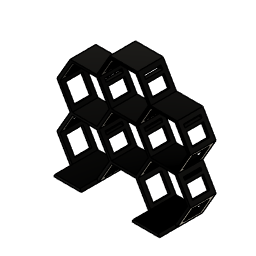
Estande v1 (Autodesk Fusion 360 design; units mm, degrees)
Autodesk Fusion 360 part; units mm, degrees
sketch "Sketch1" plane through (0, 0, 0) normal (0, 1, 0) x (1, 0, 0)
  line L0 (28.8675, 0) -> (14.4338, 25)
  line L1 (14.4338, 25) -> (-14.4338, 25)
  line L2 (-14.4338, 25) -> (-28.8675, 0)
  line L3 (-28.8675, 0) -> (-14.4338, -25)
  line L4 (-14.4338, -25) -> (14.4338, -25)
  line L5 (14.4338, -25) -> (28.8675, 0)
  line L6 (-125, -81) -> (125, -81)
  line L7 (125, -81) -> (125, 67)
  line L8 (125, 67) -> (-125, 67)
  line L9 (-125, 67) -> (-125, -81)
  line L10 (60.3331, 1.5) -> (74.7669, 26.5)
  line L11 (74.7669, 26.5) -> (60.3331, 51.5)
  line L12 (60.3331, 51.5) -> (31.4656, 51.5)
  line L13 (31.4656, 51.5) -> (17.0318, 26.5)
  line L14 (17.0318, 26.5) -> (31.4656, 1.5)
  line L15 (31.4656, 1.5) -> (60.3331, 1.5)
  line L16 (0, 0) -> (45.8993, 26.5) construction
  line L17 (0, 0) -> (0, 25) construction
  line L18 (14.4338, 78) -> (-14.4338, 78)
  line L19 (-14.4338, 78) -> (-28.8675, 53)
  line L20 (-28.8675, 53) -> (-14.4338, 28)
  line L21 (-14.4338, 28) -> (14.4338, 28)
  line L22 (28.8675, 53) -> (14.4338, 78)
  line L23 (14.4338, 28) -> (28.8675, 53)
  line L24 (-60.3331, 51.5) -> (-74.7669, 26.5)
  line L25 (-74.7669, 26.5) -> (-60.3331, 1.5)
  line L26 (-60.3331, 1.5) -> (-31.4656, 1.5)
  line L27 (-31.4656, 1.5) -> (-17.0318, 26.5)
  line L28 (-31.4656, 51.5) -> (-60.3331, 51.5)
  line L29 (-17.0318, 26.5) -> (-31.4656, 51.5)
  line L30 (-74.7669, -26.5) -> (-60.3331, -51.5)
  line L31 (-60.3331, -51.5) -> (-31.4656, -51.5)
  line L32 (-31.4656, -51.5) -> (-17.0318, -26.5)
  line L33 (-17.0318, -26.5) -> (-31.4656, -1.5)
  line L34 (-60.3331, -1.5) -> (-74.7669, -26.5)
  line L35 (-31.4656, -1.5) -> (-60.3331, -1.5)
  line L36 (-14.4338, -78) -> (14.4338, -78)
  line L37 (14.4338, -78) -> (28.8675, -53)
  line L38 (28.8675, -53) -> (14.4338, -28)
  line L39 (14.4338, -28) -> (-14.4338, -28)
  line L40 (-28.8675, -53) -> (-14.4338, -78)
  line L41 (-14.4338, -28) -> (-28.8675, -53)
  line L42 (60.3331, -51.5) -> (74.7669, -26.5)
  line L43 (74.7669, -26.5) -> (60.3331, -1.5)
  line L44 (60.3331, -1.5) -> (31.4656, -1.5)
  line L45 (31.4656, -1.5) -> (17.0318, -26.5)
  line L46 (31.4656, -51.5) -> (60.3331, -51.5)
  line L47 (17.0318, -26.5) -> (31.4656, -51.5)
  line L48 (0, -78) -> (0, -81) construction
  line L49 (125, 54.5) -> (-125, 54.5)
  line L50 (-62.0652, 54.5) -> (-78.231, 26.5)
  line L51 (-78.231, 26.5) -> (-62.7147, -0.375)
  line L52 (-62.7147, -0.375) -> (-78.231, -27.25)
  line L53 (-78.231, -27.25) -> (-62.7147, -54.125)
  line L54 (-62.7147, -54.125) -> (-31.6821, -54.125)
  line L55 (-31.6821, -54.125) -> (-16.1658, -81)
  line L56 (62.0652, 54.5) -> (78.231, 26.5)
  line L57 (78.231, 26.5) -> (62.7147, -0.375)
  line L58 (62.7147, -0.375) -> (78.231, -27.25)
  line L59 (78.231, -27.25) -> (62.7147, -54.125)
  line L60 (62.7147, -54.125) -> (31.6821, -54.125)
  line L61 (31.6821, -54.125) -> (16.1658, -81)
  line L62 (-28.8675, 53) -> (-29.7335, 54.5)
  line L63 (28.8675, 53) -> (29.7335, 54.5)
  point P0 (45.8993, 26.5)
  dimension "d3" = 50
  dimension "d4" = 60
  dimension "d5" = 3
  dimension "d6" = 148
  dimension "d7" = 250
  dimension "d9" = 360
  dimension "d10" = 3
  dimension "d11" = 3
  dimension "d12" = 3
  dimension "d14" = 3
  constraint coincident L16.start L17.start
  constraint horizontal L6
  constraint perpendicular L6 L7
  constraint perpendicular L7 L8
  constraint vertical L9
  constraint horizontal L4
  constraint horizontal L15
  constraint equal L0 L14
  constraint coincident P0 L16.end
  constraint midpoint L1 L17.end
  constraint midpoint L36 L48.start
  constraint midpoint L6 L48.end
  constraint vertical L48
  constraint coincident L7 L49.start
  constraint coincident L9 L49.end
  constraint perpendicular L9 L49
  constraint coincident L49 L50.start
  constraint parallel L49 L54
  constraint coincident L6 L55.end
  constraint parallel L53 L55
  constraint parallel L40 L55
  constraint parallel L34 L52
  constraint parallel L25 L51
  constraint parallel L24 L50
  constraint equal L54 L55
  constraint equal L53 L54
  constraint equal L52 L53
  constraint equal L51 L52
  constraint symmetric L17 L50.start L56.start
  constraint symmetric L17 L50.end L56.end
  constraint symmetric L17 L51.end L57.end
  constraint symmetric L17 L52.end L58.end
  constraint symmetric L17 L53.end L59.end
  constraint symmetric L17 L54.end L60.end
  constraint symmetric L17 L55.end L61.end
  constraint coincident L49 L62.end
  constraint parallel L20 L62
  constraint coincident L49 L63.end
  constraint parallel L23 L63
  measures "d3" distance of L1 L4
  measures "d4" angle of L16 L17
  measures "d5" distance of L0 L14
  measures "d6" distance of L6 L8
  measures "d7" distance of L6.start L6.end
  measures "d10" distance of L6 L36
  measures "d11" distance of L28 L49
  measures "d12" distance of L24 L50
  measures "d14" distance of L25 L51
extrude "Extrude1" add sketch "Sketch1" against normal blind 30 contours L6 L20 L21 L23 L49 L50 L51 L52 L53 L54 L55 L56 L57 L58 L59 L60 L61 L62 L63
sketch "Sketch2" plane through (70.4728, 0, 40.6875) normal (0.866025, 0, 0.5) x (0, 1, 0)
  line L0 (0, -15.5163) -> (0, 15.5163)
  line L1 (0, 15.5163) -> (-30, 15.5163)
  line L2 (-30, 15.5163) -> (-30, -15.5163)
  line L3 (-30, -15.5163) -> (0, -15.5163)
  line L4 (-25, -10.5163) -> (-5, -10.5163)
  line L5 (-5, -10.5163) -> (-5, 10.5163)
  line L6 (-5, 10.5163) -> (-25, 10.5163)
  line L7 (-25, 10.5163) -> (-25, -10.5163)
  line L8 (0, 31.0326) -> (0, 62.0652)
  line L9 (0, 62.0652) -> (-30, 62.0652)
  line L10 (-30, 62.0652) -> (-30, 31.0326)
  line L11 (-30, 31.0326) -> (0, 31.0326)
  line L12 (0, -62.0652) -> (0, -31.0326)
  line L13 (0, -31.0326) -> (-30, -31.0326)
  line L14 (-30, -31.0326) -> (-30, -62.0652)
  line L15 (-30, -62.0652) -> (0, -62.0652)
  line L16 (-25, -57.0652) -> (-5, -57.0652)
  line L17 (-5, -57.0652) -> (-5, -36.0326)
  line L18 (-5, -36.0326) -> (-25, -36.0326)
  line L19 (-25, -36.0326) -> (-25, -57.0652)
  line L20 (-25, 36.0326) -> (-5, 36.0326)
  line L21 (-5, 36.0326) -> (-5, 57.0652)
  line L22 (-5, 57.0652) -> (-25, 57.0652)
  line L23 (-25, 57.0652) -> (-25, 36.0326)
  dimension "d17" = -5
  dimension "d18" = -5
  dimension "d19" = -5
extrude "Extrude2" cut sketch "Sketch2" against normal blind 170 contours L4 L5 L6 L7 | L16 L17 L18 L19 | L20 L21 L22 L23
mirror "Mirror1" about plane through (0, 0, 0) normal (1, 0, 0) of "Extrude2"
sketch "Sketch3" plane through (0, -30, 0) normal (0, -1, 0) x (1, 0, 0)
  line L0 (-17.0318, -26.5) -> (-31.4656, -51.5)
  line L1 (-31.4656, -51.5) -> (-60.3331, -51.5)
  line L2 (-60.3331, -51.5) -> (-74.7669, -26.5)
  line L3 (-74.7669, -26.5) -> (-60.3331, -1.5)
  line L4 (-60.3331, -1.5) -> (-31.4656, -1.5)
  line L5 (-31.4656, -1.5) -> (-17.0318, -26.5)
  line L6 (31.4656, -1.5) -> (60.3331, -1.5)
  line L7 (60.3331, -1.5) -> (74.7669, -26.5)
  line L8 (74.7669, -26.5) -> (60.3331, -51.5)
  line L9 (60.3331, -51.5) -> (31.4656, -51.5)
  line L10 (31.4656, -51.5) -> (17.0318, -26.5)
  line L11 (17.0318, -26.5) -> (31.4656, -1.5)
  line L12 (17.0318, 26.5) -> (31.4656, 51.5)
  line L13 (31.4656, 51.5) -> (60.3331, 51.5)
  line L14 (60.3331, 51.5) -> (74.7669, 26.5)
  line L15 (74.7669, 26.5) -> (60.3331, 1.5)
  line L16 (60.3331, 1.5) -> (31.4656, 1.5)
  line L17 (31.4656, 1.5) -> (17.0318, 26.5)
  line L18 (-14.4338, 28) -> (-28.8675, 53)
  line L19 (-28.8675, 53) -> (-14.4338, 78)
  line L20 (-14.4338, 78) -> (14.4338, 78)
  line L21 (14.4338, 78) -> (28.8675, 53)
  line L22 (28.8675, 53) -> (14.4338, 28)
  line L23 (14.4338, 28) -> (-14.4338, 28)
  line L24 (-31.4656, 1.5) -> (-60.3331, 1.5)
  line L25 (-60.3331, 1.5) -> (-74.7669, 26.5)
  line L26 (-74.7669, 26.5) -> (-60.3331, 51.5)
  line L27 (-60.3331, 51.5) -> (-31.4656, 51.5)
  line L28 (-31.4656, 51.5) -> (-17.0318, 26.5)
  line L29 (-17.0318, 26.5) -> (-31.4656, 1.5)
  line L30 (14.4338, 25) -> (28.8675, 0)
  line L31 (28.8675, 0) -> (14.4338, -25)
  line L32 (14.4338, -25) -> (-14.4338, -25)
  line L33 (-14.4338, -25) -> (-28.8675, 0)
  line L34 (-28.8675, 0) -> (-14.4338, 25)
  line L35 (-14.4338, 25) -> (14.4338, 25)
  line L36 (29.7335, -54.5) -> (62.0652, -54.5)
  line L37 (62.0652, -54.5) -> (78.231, -26.5)
  line L38 (78.231, -26.5) -> (62.7147, 0.375)
  line L39 (62.7147, 0.375) -> (78.231, 27.25)
  line L40 (78.231, 27.25) -> (62.7147, 54.125)
  line L41 (62.7147, 54.125) -> (31.6821, 54.125)
  line L42 (31.6821, 54.125) -> (16.1658, 81)
  line L43 (16.1658, 81) -> (-16.1658, 81)
  line L44 (-16.1658, 81) -> (-31.6821, 54.125)
  line L45 (-31.6821, 54.125) -> (-62.7147, 54.125)
  line L46 (-62.7147, 54.125) -> (-78.231, 27.25)
  line L47 (-78.231, 27.25) -> (-62.7147, 0.375)
  line L48 (-62.7147, 0.375) -> (-78.231, -26.5)
  line L49 (-78.231, -26.5) -> (-62.0652, -54.5)
  line L50 (-62.0652, -54.5) -> (-29.7335, -54.5)
  line L51 (-29.7335, -54.5) -> (-14.4338, -28)
  line L52 (-14.4338, -28) -> (14.4338, -28)
  line L53 (14.4338, -28) -> (29.7335, -54.5)
  line L54 (60.3331, -51.5) -> (62.0652, -54.5)
  line L55 (31.4656, -51.5) -> (29.7335, -54.5)
  line L56 (-60.3331, -51.5) -> (-62.0652, -54.5)
  line L57 (-31.4656, -51.5) -> (-29.7335, -54.5)
  constraint coincident L8.end L9.start
  constraint coincident L36.end L37.start
  constraint coincident L9.end L10.start
  constraint coincident L36.start L53.end
  constraint coincident L1.end L2.start
  constraint coincident L49.end L50.start
  constraint coincident L0.end L1.start
  constraint coincident L50.end L51.start
extrude "Extrude3" add sketch "Sketch3" along normal blind 20 contours L1 L50 L56 L57 | L9 L36 L54 L55
sketch "Sketch4" plane through (0, 0, 0) normal (0, 1, 0) x (-1, 0, 0)
  line L0 (28.8675, 53) -> (14.4338, 28)
  line L1 (14.4338, 28) -> (-14.4338, 28)
  line L2 (-14.4338, 28) -> (-28.8675, 53)
  line L3 (-28.8675, 53) -> (-14.4338, 78)
  line L4 (-14.4338, 78) -> (14.4338, 78)
  line L5 (14.4338, 78) -> (28.8675, 53)
  line L6 (-60.3331, -1.5) -> (-31.4656, -1.5)
  line L7 (-31.4656, -1.5) -> (-17.0318, -26.5)
  line L8 (-17.0318, -26.5) -> (-31.4656, -51.5)
  line L9 (-31.4656, -51.5) -> (-60.3331, -51.5)
  line L10 (-60.3331, -51.5) -> (-74.7669, -26.5)
  line L11 (-74.7669, -26.5) -> (-60.3331, -1.5)
  line L12 (-31.4656, 51.5) -> (-17.0318, 26.5)
  line L13 (-17.0318, 26.5) -> (-31.4656, 1.5)
  line L14 (-31.4656, 1.5) -> (-60.3331, 1.5)
  line L15 (-60.3331, 1.5) -> (-74.7669, 26.5)
  line L16 (-74.7669, 26.5) -> (-60.3331, 51.5)
  line L17 (-60.3331, 51.5) -> (-31.4656, 51.5)
  line L18 (31.4656, -51.5) -> (17.0318, -26.5)
  line L19 (17.0318, -26.5) -> (31.4656, -1.5)
  line L20 (31.4656, -1.5) -> (60.3331, -1.5)
  line L21 (60.3331, -1.5) -> (74.7669, -26.5)
  line L22 (74.7669, -26.5) -> (60.3331, -51.5)
  line L23 (60.3331, -51.5) -> (31.4656, -51.5)
  line L24 (60.3331, 1.5) -> (31.4656, 1.5)
  line L25 (31.4656, 1.5) -> (17.0318, 26.5)
  line L26 (17.0318, 26.5) -> (31.4656, 51.5)
  line L27 (31.4656, 51.5) -> (60.3331, 51.5)
  line L28 (60.3331, 51.5) -> (74.7669, 26.5)
  line L29 (74.7669, 26.5) -> (60.3331, 1.5)
  line L30 (-28.8675, 0) -> (-14.4338, 25)
  line L31 (-14.4338, 25) -> (14.4338, 25)
  line L32 (14.4338, 25) -> (28.8675, 0)
  line L33 (28.8675, 0) -> (14.4338, -25)
  line L34 (14.4338, -25) -> (-14.4338, -25)
  line L35 (-14.4338, -25) -> (-28.8675, 0)
  line L36 (14.4338, -28) -> (29.7335, -54.5)
  line L37 (29.7335, -54.5) -> (62.0652, -54.5)
  line L38 (62.0652, -54.5) -> (78.231, -26.5)
  line L39 (78.231, -26.5) -> (62.7147, 0.375)
  line L40 (62.7147, 0.375) -> (78.231, 27.25)
  line L41 (78.231, 27.25) -> (62.7147, 54.125)
  line L42 (62.7147, 54.125) -> (31.6821, 54.125)
  line L43 (31.6821, 54.125) -> (16.1658, 81)
  line L44 (16.1658, 81) -> (-16.1658, 81)
  line L45 (-16.1658, 81) -> (-31.6821, 54.125)
  line L46 (-31.6821, 54.125) -> (-62.7147, 54.125)
  line L47 (-62.7147, 54.125) -> (-78.231, 27.25)
  line L48 (-78.231, 27.25) -> (-62.7147, 0.375)
  line L49 (-62.7147, 0.375) -> (-78.231, -26.5)
  line L50 (-78.231, -26.5) -> (-62.0652, -54.5)
  line L51 (-62.0652, -54.5) -> (-29.7335, -54.5)
  line L52 (-29.7335, -54.5) -> (-14.4338, -28)
  line L53 (-14.4338, -28) -> (14.4338, -28)
  line L54 (-66.9005, 46.875) -> (-25.3312, 46.875)
  line L55 (-68.6325, 43.875) -> (-23.5992, 43.875)
  line L56 (-22.5167, 70) -> (22.5167, 70)
  line L57 (20.7846, 73) -> (-20.7846, 73)
  line L58 (25.3312, 46.875) -> (66.9005, 46.875)
  line L59 (68.6325, 43.875) -> (23.5992, 43.875)
  line L60 (20.7846, 20) -> (-20.7846, 20)
  line L61 (22.5167, 17) -> (-22.5167, 17)
  line L62 (-25.1147, -6.5) -> (-66.684, -6.5)
  line L63 (-68.416, -9.5) -> (-23.3827, -9.5)
  line L64 (66.684, -6.5) -> (25.1147, -6.5)
  line L65 (23.3827, -9.5) -> (68.416, -9.5)
  dimension "d35" = 3
  dimension "d36" = 5
  constraint coincident L47 L54.start
  constraint coincident L2 L54.end
  constraint horizontal L54
  constraint coincident L47 L55.start
  constraint coincident L2 L55.end
  constraint horizontal L55
  constraint coincident L45 L56.start
  constraint coincident L43 L56.end
  constraint horizontal L56
  constraint coincident L43 L57.start
  constraint coincident L45 L57.end
  constraint parallel L56 L57
  constraint equal L54 L57
  constraint equal L55 L56
  constraint coincident L0 L58.start
  constraint coincident L41 L58.end
  constraint horizontal L58
  constraint coincident L41 L59.start
  constraint coincident L0 L59.end
  constraint parallel L58 L59
  constraint equal L57 L58
  constraint equal L56 L59
  constraint coincident L25 L60.start
  constraint coincident L13 L60.end
  constraint horizontal L60
  constraint coincident L25 L61.start
  constraint coincident L13 L61.end
  constraint parallel L60 L61
  constraint coincident L35 L62.start
  constraint coincident L49 L62.end
  constraint parallel L61 L62
  constraint coincident L49 L63.start
  constraint coincident L35 L63.end
  constraint parallel L62 L63
  constraint coincident L39 L64.start
  constraint coincident L33 L64.end
  constraint parallel L63 L64
  constraint coincident L33 L65.start
  constraint coincident L39 L65.end
  constraint parallel L64 L65
  constraint equal L58 L64
  constraint equal L59 L65
  constraint equal L57 L60
  constraint equal L56 L61
  constraint equal L54 L62
  constraint equal L55 L63
  measures "d35" distance of L56 L57
  measures "d36" distance of L4 L57
extrude "Extrude6" add sketch "Sketch4" against normal blind 3 contours L3 L5 L56 L57 | L26 L28 L58 L59 | L12 L16 L54 L55 | L30 L32 L60 L61 | L19 L21 L64 L65 | L7 L11 L62 L63
extrude "Extrude4" add sketch "Sketch4" against normal up to surface (30 mm away) contours L0 L26 L58 L59 | L5 L43 L56 L57 | L3 L45 L56 L57 | L28 L41 L58 L59 | L2 L12 L54 L55 | L25 L32 L60 L61 | L16 L47 L54 L55 | L13 L30 L60 L61 | L21 L39 L64 L65 | L19 L33 L64 L65 | L7 L35 L62 L63 | L11 L49 L62 L63
named bodies: "Body2 (1)", "Body2 (2)"
